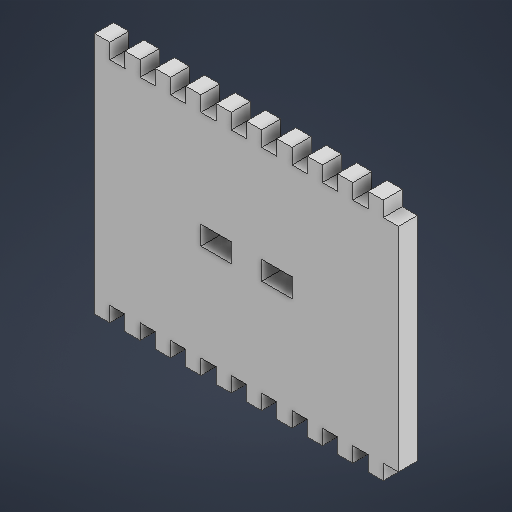
# Autodesk Inventor part: pitahaya4
Saved by Autodesk Inventor 2026.3 (Build 303398000, 398)
## iProperties
Created: 2026-09-15
Part Number: pitahaya4
Material: Generic
Document SubType Name: Modeling
Designer: micha
Density: 1 g/cm^3
Appearance: Default
Author: micha
Autodesk Inventor part; units mm, degrees
ref_plane "YZ Plane" through (0, 0, 0) normal (1, 0, 0) x (0, 1, 0)
ref_plane "XZ Plane" through (0, 0, 0) normal (0, 1, 0) x (-1, 0, 0)
ref_plane "XY Plane" through (0, 0, 0) normal (0, 0, 1) x (1, 0, 0)
sketch "Sketch1" plane through (0, 0, 0) normal (0, 0, 1) x (1, 0, 0)
  line L0 (0, 8.7149) -> (0, -8.7149) construction
  line L1 (-12.4402, 0) -> (12.4402, 0) construction
  line L2 (-20, 14) -> (20, 14) construction
  line L3 (20, 14) -> (20, -14) construction
  line L4 (20, -14) -> (-20, -14) construction
  line L5 (-20, -14) -> (-20, 14) construction
  line L6 (-6, 1.25) -> (-2, 1.25)
  line L7 (-2, 1.25) -> (-2, -1.25)
  line L8 (-2, -1.25) -> (-6, -1.25)
  line L9 (-6, -1.25) -> (-6, 1.25)
  line L10 (2, 1.25) -> (6, 1.25)
  line L11 (6, 1.25) -> (6, -1.25)
  line L12 (6, -1.25) -> (2, -1.25)
  line L13 (2, -1.25) -> (2, 1.25)
  line L14 (-20, 14) -> (-20, 16)
  line L15 (-20, 16) -> (-18, 16)
  line L16 (-18, 16) -> (-18, 14)
  line L17 (-16, 14) -> (-16, 16)
  line L18 (-16, 16) -> (-14, 16)
  line L19 (-14, 16) -> (-14, 14)
  line L20 (-12, 14) -> (-12, 16)
  line L21 (-12, 16) -> (-10, 16)
  line L22 (-10, 16) -> (-10, 14)
  line L23 (-8, 14) -> (-8, 16)
  line L24 (-8, 16) -> (-6, 16)
  line L25 (-6, 16) -> (-6, 14)
  line L26 (-4, 14) -> (-4, 16)
  line L27 (-4, 16) -> (-2, 16)
  line L28 (-2, 16) -> (-2, 14)
  line L29 (0, 14) -> (0, 16)
  line L30 (0, 16) -> (2, 16)
  line L31 (2, 16) -> (2, 14)
  line L32 (4, 14) -> (4, 16)
  line L33 (4, 16) -> (6, 16)
  line L34 (6, 16) -> (6, 14)
  line L35 (8, 14) -> (8, 16)
  line L36 (8, 16) -> (10, 16)
  line L37 (10, 16) -> (10, 14)
  line L38 (12, 14) -> (12, 16)
  line L39 (12, 16) -> (14, 16)
  line L40 (14, 16) -> (14, 14)
  line L41 (16, 14) -> (16, 16)
  line L42 (16, 16) -> (18, 16)
  line L43 (18, 16) -> (18, 14)
  line L44 (-10, 14) -> (-8, 14)
  line L45 (-14, 14) -> (-12, 14)
  line L46 (-18, 14) -> (-16, 14)
  line L47 (-6, 14) -> (-4, 14)
  line L48 (-2, 14) -> (0, 14)
  line L49 (2, 14) -> (4, 14)
  line L50 (6, 14) -> (8, 14)
  line L51 (10, 14) -> (12, 14)
  line L52 (14, 14) -> (16, 14)
  line L53 (-20, -14) -> (-20, -16)
  line L54 (-20, -16) -> (-18, -16)
  line L55 (-18, -16) -> (-18, -14)
  line L56 (-16, -14) -> (-16, -16)
  line L57 (-14, -16) -> (-14, -14)
  line L58 (-16, -16) -> (-14, -16)
  line L59 (-12, -14) -> (-12, -16)
  line L60 (-10, -16) -> (-10, -14)
  line L61 (-12, -16) -> (-10, -16)
  line L62 (-8, -14) -> (-8, -16)
  line L63 (-6, -16) -> (-6, -14)
  line L64 (-8, -16) -> (-6, -16)
  line L65 (-4, -14) -> (-4, -16)
  line L66 (-2, -16) -> (-2, -14)
  line L67 (-4, -16) -> (-2, -16)
  line L68 (0, -14) -> (0, -16)
  line L69 (2, -16) -> (2, -14)
  line L70 (0, -16) -> (2, -16)
  line L71 (4, -14) -> (4, -16)
  line L72 (6, -16) -> (6, -14)
  line L73 (4, -16) -> (6, -16)
  line L74 (8, -14) -> (8, -16)
  line L75 (10, -16) -> (10, -14)
  line L76 (8, -16) -> (10, -16)
  line L77 (12, -14) -> (12, -16)
  line L78 (14, -16) -> (14, -14)
  line L79 (12, -16) -> (14, -16)
  line L80 (16, -14) -> (16, -16)
  line L81 (18, -16) -> (18, -14)
  line L82 (16, -16) -> (18, -16)
  line L83 (-18, -14) -> (-16, -14)
  line L84 (-14, -14) -> (-12, -14)
  line L85 (-10, -14) -> (-8, -14)
  line L86 (-6, -14) -> (-4, -14)
  line L87 (-2, -14) -> (0, -14)
  line L88 (2, -14) -> (4, -14)
  line L89 (6, -14) -> (8, -14)
  line L90 (10, -14) -> (12, -14)
  line L91 (14, -14) -> (16, -14)
  line L92 (18, -14) -> (20, -14)
  line L93 (18, 14) -> (20, 14)
  line L94 (20, 14) -> (20, -14)
  line L95 (-20, 14) -> (-20, -14)
  point P0 (0, 0)
  point P1 (0, 0)
  dimension "d0" = 4
  dimension "d1" = 4
  dimension "d2" = 4
  dimension "d3" = 2.5
  dimension "d4" = 28
  dimension "d5" = 40
  dimension "d10" = 2
  dimension "d11" = 2
  dimension "d14" = 4
  dimension "d19" = 2
  dimension "d22" = 4
  constraints: 192 end point, 15 collinear, 11 perpendicular, 8 horizontal, 6 parallel, 4 point on line, 3 coincident, 3 vertical, 2 horizontal alignment, 2 midpoint, 1 vertical alignment, 130 other
  measures "d0" distance of L6.start L6.end
  measures "d1" distance of L10.start L10.end
  measures "d2" distance between parallel lines of L13 L7
  measures "d3" distance of L8.end L6.start
  measures "d4" distance of L4.end L2.start
  measures "d5" distance of L3.end L4.end
  measures "d10" distance of L2.start L14.end
  measures "d11" distance of L14.end L15.end
  measures "d14" distance of L2.start L17.start
  measures "d19" distance of L4.end L53.end
  measures "d22" distance of L4.end L56.start
extrude "Extrusion1" add sketch "Sketch1" along normal mid plane 2.5
body "Solid1"
